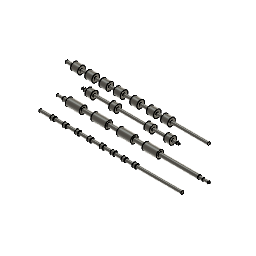
Salvage v1 (Autodesk Fusion 360 design; units mm, degrees)
Autodesk Fusion 360 part; units mm, degrees
sketch "Sketch1" plane through (0, 0, 0) normal (0, 1, 0) x (1, 0, 0) in component "axle1"
  line L0 (-152.5538, -2) -> (147.4462, -2)
  line L1 (147.4462, -2) -> (147.4462, -5)
  line L2 (147.4462, -5) -> (-152.5538, -5)
  line L3 (-152.5538, -5) -> (-152.5538, -2)
  line L4 (-136.5538, -5) -> (-121.5538, -5)
  line L5 (-121.5538, -5) -> (-121.5538, -10)
  line L6 (-121.5538, -10) -> (-136.5538, -10)
  line L7 (-136.5538, -10) -> (-136.5538, -5)
  line L8 (-106.5538, -5) -> (-91.5538, -5)
  line L9 (-91.5538, -5) -> (-91.5538, -10)
  line L10 (-91.5538, -10) -> (-106.5538, -10)
  line L11 (-106.5538, -10) -> (-106.5538, -5)
  line L12 (-76.5538, -5) -> (-61.5538, -5)
  line L13 (-61.5538, -5) -> (-61.5538, -10)
  line L14 (-61.5538, -10) -> (-76.5538, -10)
  line L15 (-76.5538, -10) -> (-76.5538, -5)
  line L16 (-46.5538, -5) -> (-31.5538, -5)
  line L17 (-31.5538, -5) -> (-31.5538, -10)
  line L18 (-31.5538, -10) -> (-46.5538, -10)
  line L19 (-46.5538, -10) -> (-46.5538, -5)
  line L20 (-11.5538, -5) -> (3.4462, -5)
  line L21 (3.4462, -5) -> (3.4462, -10)
  line L22 (3.4462, -10) -> (-11.5538, -10)
  line L23 (-11.5538, -10) -> (-11.5538, -5)
  line L24 (23.4462, -5) -> (38.4462, -5)
  line L25 (38.4462, -5) -> (38.4462, -10)
  line L26 (38.4462, -10) -> (23.4462, -10)
  line L27 (23.4462, -10) -> (23.4462, -5)
  line L28 (53.4462, -5) -> (68.4462, -5)
  line L29 (68.4462, -5) -> (68.4462, -10)
  line L30 (68.4462, -10) -> (53.4462, -10)
  line L31 (53.4462, -10) -> (53.4462, -5)
  dimension "d1" = 16
  dimension "d2" = 3
  dimension "d3" = 15
  dimension "d4" = 5
  dimension "d5" = 300
  dimension "d6" = 15
  dimension "d7" = 15
  dimension "d8" = 15
  dimension "d9" = 20
  dimension "d10" = 20
  dimension "d11" = 15
  constraint horizontal L0
  constraint vertical L1
  constraint horizontal L2
  constraint vertical L3
  constraint horizontal L4
  constraint vertical L5
  constraint horizontal L6
  constraint vertical L7
  constraint coincident L2 L4.start
  constraint horizontal L8
  constraint vertical L9
  constraint horizontal L10
  constraint vertical L11
  constraint coincident L2 L8.start
  constraint horizontal L12
  constraint vertical L13
  constraint horizontal L14
  constraint vertical L15
  constraint coincident L2 L12.start
  constraint horizontal L16
  constraint vertical L17
  constraint horizontal L18
  constraint vertical L19
  constraint coincident L2 L16.start
  constraint horizontal L20
  constraint vertical L21
  constraint horizontal L22
  constraint vertical L23
  constraint coincident L2 L20.start
  constraint horizontal L24
  constraint vertical L25
  constraint horizontal L26
  constraint vertical L27
  constraint coincident L2 L24.start
  constraint horizontal L28
  constraint vertical L29
  constraint horizontal L30
  constraint vertical L31
  constraint coincident L2 L28.start
  constraint equal L26 L30
  constraint equal L22 L26
  constraint equal L18 L22
  constraint equal L14 L18
  constraint equal L10 L14
  constraint equal L6 L10
  constraint equal L7 L11
  constraint equal L11 L15
  constraint equal L15 L19
  constraint equal L19 L23
  constraint equal L23 L27
  constraint equal L27 L31
  measures "d1" distance of L2.end L4.start
  measures "d2" distance of L0.start L2.end
  measures "d3" distance of L5.end L6.end
  measures "d4" distance of L4.start L6.end
  measures "d5" distance of L1.end L2.end
  measures "d6" distance of L4.end L8.start
  measures "d7" distance of L8.end L12.start
  measures "d8" distance of L12.end L16.start
  measures "d9" distance of L16.end L20.start
  measures "d10" distance of L20.end L24.start
  measures "d11" distance of L24.end L28.start
revolve "Revolve1" add sketch "Sketch1" angle 360 about axis through (-152.5538, 0, 2) along (1, 0, 0) makes body 1 in component "axle1"
sketch "Sketch1 (2)" plane through (0, 0, 0) normal (0, 1, 0) x (1, 0, 0) in component "axle2"
  line L0 (-92.2895, -1.3003) -> (207.7105, -1.3003)
  line L1 (207.7105, -1.3003) -> (207.7105, -4.3003)
  line L2 (207.7105, -4.3003) -> (-92.2895, -4.3003)
  line L3 (-92.2895, -4.3003) -> (-92.2895, -1.3003)
  line L4 (-67.2895, -4.3003) -> (-61.2895, -4.3003)
  line L5 (-61.2895, -4.3003) -> (-61.2895, -5.8003)
  line L6 (-61.2895, -5.8003) -> (-67.2895, -5.8003)
  line L7 (-67.2895, -5.8003) -> (-67.2895, -4.3003)
  line L8 (-41.2895, -4.3003) -> (-35.2895, -4.3003)
  line L9 (-35.2895, -4.3003) -> (-35.2895, -5.8003)
  line L10 (-35.2895, -5.8003) -> (-41.2895, -5.8003)
  line L11 (-41.2895, -5.8003) -> (-41.2895, -4.3003)
  line L12 (-15.2895, -4.3003) -> (-9.2895, -4.3003)
  line L13 (-9.2895, -4.3003) -> (-9.2895, -5.8003)
  line L14 (-9.2895, -5.8003) -> (-15.2895, -5.8003)
  line L15 (-15.2895, -5.8003) -> (-15.2895, -4.3003)
  line L16 (10.7105, -4.3003) -> (16.7105, -4.3003)
  line L17 (16.7105, -4.3003) -> (16.7105, -5.8003)
  line L18 (16.7105, -5.8003) -> (10.7105, -5.8003)
  line L19 (10.7105, -5.8003) -> (10.7105, -4.3003)
  line L20 (36.7105, -4.3003) -> (42.7105, -4.3003)
  line L21 (42.7105, -4.3003) -> (42.7105, -5.8003)
  line L22 (42.7105, -5.8003) -> (36.7105, -5.8003)
  line L23 (36.7105, -5.8003) -> (36.7105, -4.3003)
  line L24 (59.7105, -4.3003) -> (65.7105, -4.3003)
  line L25 (65.7105, -4.3003) -> (65.7105, -5.8003)
  line L26 (65.7105, -5.8003) -> (59.7105, -5.8003)
  line L27 (59.7105, -5.8003) -> (59.7105, -4.3003)
  line L28 (82.7105, -4.3003) -> (88.7105, -4.3003)
  line L29 (88.7105, -4.3003) -> (88.7105, -5.8003)
  line L30 (88.7105, -5.8003) -> (82.7105, -5.8003)
  line L31 (82.7105, -5.8003) -> (82.7105, -4.3003)
  line L32 (105.7105, -4.3003) -> (111.7105, -4.3003)
  line L33 (111.7105, -4.3003) -> (111.7105, -5.8003)
  line L34 (111.7105, -5.8003) -> (105.7105, -5.8003)
  line L35 (105.7105, -5.8003) -> (105.7105, -4.3003)
  dimension "d13" = 3
  dimension "d14" = 300
  dimension "d15" = 25
  dimension "d16" = 1.5
  dimension "d17" = 6
  dimension "d18" = 20
  dimension "d19" = 20
  dimension "d20" = 20
  dimension "d21" = 20
  dimension "d22" = 17
  dimension "d23" = 17
  dimension "d24" = 17
  constraint horizontal L0
  constraint vertical L1
  constraint horizontal L2
  constraint vertical L3
  constraint horizontal L4
  constraint vertical L5
  constraint horizontal L6
  constraint vertical L7
  constraint coincident L2 L4.start
  constraint horizontal L8
  constraint vertical L9
  constraint horizontal L10
  constraint vertical L11
  constraint coincident L2 L8.start
  constraint horizontal L12
  constraint vertical L13
  constraint horizontal L14
  constraint vertical L15
  constraint coincident L2 L12.start
  constraint horizontal L16
  constraint vertical L17
  constraint horizontal L18
  constraint vertical L19
  constraint coincident L2 L16.start
  constraint horizontal L20
  constraint vertical L21
  constraint horizontal L22
  constraint vertical L23
  constraint coincident L2 L20.start
  constraint horizontal L24
  constraint vertical L25
  constraint horizontal L26
  constraint vertical L27
  constraint coincident L2 L24.start
  constraint horizontal L28
  constraint vertical L29
  constraint horizontal L30
  constraint vertical L31
  constraint coincident L2 L28.start
  constraint horizontal L32
  constraint vertical L33
  constraint horizontal L34
  constraint vertical L35
  constraint coincident L2 L32.start
  constraint equal L6 L10
  constraint equal L10 L14
  constraint equal L14 L18
  constraint equal L18 L22
  constraint equal L22 L26
  constraint equal L26 L30
  constraint equal L30 L34
  constraint equal L31 L35
  constraint equal L27 L31
  constraint equal L23 L27
  constraint equal L19 L23
  constraint equal L15 L19
  constraint equal L11 L15
  constraint equal L7 L11
  measures "d13" distance of L0.start L2.end
  measures "d14" distance of L1.end L2.end
  measures "d15" distance of L2.end L4.start
  measures "d16" distance of L4.start L6.end
  measures "d17" distance of L5.end L6.end
  measures "d18" distance of L4.end L8.start
  measures "d19" distance of L8.end L12.start
  measures "d20" distance of L12.end L16.start
  measures "d21" distance of L16.end L20.start
  measures "d22" distance of L20.end L24.start
  measures "d23" distance of L24.end L28.start
  measures "d24" distance of L28.end L32.start
revolve "Revolve1'" add sketch "Sketch1 (2)" angle 360 about axis through (-92.2895, 0, 1.3003) along (1, 0, 0) separate body makes body 2 in component "axle2"
sketch "Sketch1 (3)" plane through (0, 0, 0) normal (0, 1, 0) x (1, 0, 0) in component "axle3"
  line L0 (224.232, -5.3472) -> (-61.268, -5.3472)
  line L1 (-61.768, -4.8472) -> (-61.768, -3.6472)
  line L2 (-50.768, -5.3472) -> (-20.768, -5.3472)
  line L3 (-20.768, -5.3472) -> (-20.768, -9.1472)
  line L4 (-20.768, -9.1472) -> (-50.768, -9.1472)
  line L5 (-50.768, -9.1472) -> (-50.768, -5.3472)
  line L6 (3.232, -5.3472) -> (33.232, -5.3472)
  line L7 (33.232, -5.3472) -> (33.232, -9.1472)
  line L8 (33.232, -9.1472) -> (3.232, -9.1472)
  line L9 (3.232, -9.1472) -> (3.232, -5.3472)
  line L10 (57.232, -5.3472) -> (87.232, -5.3472)
  line L11 (87.232, -5.3472) -> (87.232, -9.1472)
  line L12 (87.232, -9.1472) -> (57.232, -9.1472)
  line L13 (57.232, -9.1472) -> (57.232, -5.3472)
  line L14 (111.232, -5.3472) -> (141.232, -5.3472)
  line L15 (141.232, -5.3472) -> (141.232, -9.1472)
  line L16 (141.232, -9.1472) -> (111.232, -9.1472)
  line L17 (111.232, -9.1472) -> (111.232, -5.3472)
  line L18 (-61.768, -3.6472) -> (-75.193, -3.6472)
  line L19 (-75.768, -3.0722) -> (-75.768, -1.3472)
  line L20 (224.232, -5.3472) -> (224.232, -1.3472)
  line L21 (224.232, -1.3472) -> (-75.768, -1.3472)
  line L22 (224.232, -4.3472) -> (232.962, -4.3472)
  line L23 (233.462, -3.8472) -> (233.462, -1.3472)
  line L24 (233.462, -1.3472) -> (224.232, -1.3472)
  line L25 (224.232, -1.3472) -> (224.232, -4.3472)
  line L26 (233.462, -3.8472) -> (244.212, -3.8472)
  line L27 (245.962, -2.8472) -> (245.962, -1.3472)
  line L28 (245.962, -1.3472) -> (233.462, -1.3472)
  line L29 (233.462, -1.3472) -> (233.462, -3.8472)
  line L30 (-75.193, -3.6472) -> (-75.768, -3.0722)
  line L31 (-61.268, -5.3472) -> (-61.768, -4.8472)
  line L32 (244.212, -3.8472) -> (245.962, -2.8472)
  line L33 (232.962, -4.3472) -> (233.462, -3.8472)
  point P0 (-61.768, -5.3472)
  point P1 (-75.768, -3.6472)
  point P2 (233.462, -4.3472)
  point P3 (245.962, -3.8472)
  dimension "d26" = 14
  dimension "d27" = 2.3
  dimension "d29" = 3.8
  dimension "d30" = 30
  dimension "d32" = 11
  dimension "d33" = 24
  dimension "d34" = 24
  dimension "d35" = 24
  dimension "d36" = 300
  dimension "d37" = 2.5
  dimension "d38" = 3
  dimension "d39" = 4
  dimension "d40" = 0.575
  dimension "d41" = 45
  dimension "d42" = 0.5
  dimension "d43" = 45
  dimension "d44" = 9.23
  dimension "d45" = 12.5
  dimension "d46" = 1.75
  dimension "d47" = 1
  dimension "d48" = 0.5
  dimension "d49" = 0.5
  constraint horizontal L0
  constraint vertical L1
  constraint horizontal L2
  constraint vertical L3
  constraint horizontal L4
  constraint vertical L5
  constraint coincident L0 L2.start
  constraint horizontal L6
  constraint vertical L7
  constraint horizontal L8
  constraint vertical L9
  constraint coincident L0 L6.start
  constraint horizontal L10
  constraint vertical L11
  constraint horizontal L12
  constraint vertical L13
  constraint coincident L0 L10.start
  constraint horizontal L14
  constraint vertical L15
  constraint horizontal L16
  constraint vertical L17
  constraint coincident L0 L14.start
  constraint horizontal L18
  constraint vertical L19
  constraint equal L12 L16
  constraint equal L8 L12
  constraint equal L4 L8
  constraint equal L5 L9
  constraint equal L13 L17
  constraint equal L9 L13
  constraint perpendicular L19 L21
  constraint horizontal L22
  constraint vertical L23
  constraint horizontal L24
  constraint vertical L25
  constraint coincident L20 L22.start
  constraint horizontal L26
  constraint vertical L27
  constraint horizontal L28
  constraint vertical L29
  constraint collinear L24 L28
  constraint collinear L21 L24
  constraint coincident P1 L18
  constraint coincident P1 L19
  constraint coincident P0 L0
  constraint coincident P0 L1
  constraint collinear L23 L29
  constraint coincident P3 L26
  constraint coincident P3 L27
  constraint coincident P2 L22
  constraint coincident P2 L23
  measures "d26" distance of L1.end P1
  measures "d27" distance of P1 L19.end
  measures "d29" distance of L2.start L4.end
  measures "d30" distance of L3.end L4.end
  measures "d32" distance of P0 L2.start
  measures "d33" distance of L2.end L6.start
  measures "d34" distance of L6.end L10.start
  measures "d35" distance of L10.end L14.start
  measures "d36" distance of L19.end L20.end
  measures "d37" distance of P3 L27.end
  measures "d38" distance of P2 L23.end
  measures "d39" distance of L20.end L0.start
  measures "d40" distance of P1 L18.end
  measures "d41" angle of L18 L30
  measures "d42" distance of P0 L0.end
  measures "d43" angle of L0 L31
  measures "d44" distance of L22.start P2
  measures "d45" distance of L23.start P3
  measures "d46" distance of P3 L26.end
  measures "d47" distance of P3 L27.start
  measures "d48" distance of P2 L22.end
  measures "d49" distance of P2 L23.start
revolve "Revolve1''" add sketch "Sketch1 (3)" angle 360 about axis through (245.962, 0, 1.3472) along (-1, 0, 0) separate body makes body 3 in component "axle3"
copy_body "CutPasteBodies1" bodies 3 removing the originals makes body 4 in component "axle3"
sketch "Sketch1 (4)" plane through (0, 0, 0) normal (1, 0, 0) x (0, 1, 0) in component "axle4"
  line L0 (-204.9118, 10.3817) -> (-8.8818, 10.3817)
  line L1 (-8.8818, 10.3817) -> (-8.8818, 12.8817)
  line L2 (-9.3818, 13.3817) -> (-204.4118, 13.3817)
  line L3 (-17.6918, 13.3817) -> (-29.2918, 13.3817)
  line L4 (-29.2918, 13.3817) -> (-29.2918, 18.2617)
  line L5 (-29.2918, 18.2617) -> (-17.6918, 18.2617)
  line L6 (-17.6918, 18.2617) -> (-17.6918, 13.3817)
  line L7 (-67.5118, 13.3817) -> (-79.1118, 13.3817)
  line L8 (-79.1118, 13.3817) -> (-79.1118, 18.2617)
  line L9 (-79.1118, 18.2617) -> (-67.5118, 18.2617)
  line L10 (-67.5118, 18.2617) -> (-67.5118, 13.3817)
  line L11 (-142.1118, 13.3817) -> (-153.7118, 13.3817)
  line L12 (-153.7118, 13.3817) -> (-153.7118, 18.2617)
  line L13 (-153.7118, 18.2617) -> (-142.1118, 18.2617)
  line L14 (-142.1118, 18.2617) -> (-142.1118, 13.3817)
  line L15 (-183.7118, 13.3817) -> (-195.3118, 13.3817)
  line L16 (-195.3118, 13.3817) -> (-195.3118, 18.2617)
  line L17 (-195.3118, 18.2617) -> (-183.7118, 18.2617)
  line L18 (-183.7118, 18.2617) -> (-183.7118, 13.3817)
  line L19 (-204.9118, 10.3817) -> (-208.9118, 10.3817)
  line L20 (-208.9118, 10.3817) -> (-208.9118, 11.6817)
  line L21 (-208.4118, 12.1817) -> (-204.9118, 12.1817)
  line L22 (-204.9118, 12.1817) -> (-204.9118, 10.3817)
  line L23 (-8.8818, 12.3817) -> (-4.8618, 12.3817)
  line L24 (-4.3618, 11.8817) -> (-4.3618, 10.3817)
  line L25 (-4.3618, 10.3817) -> (-8.8818, 10.3817)
  line L26 (-8.8818, 10.3817) -> (-8.8818, 12.3817)
  line L27 (-204.9118, 12.1817) -> (-204.9118, 12.8817)
  line L28 (-8.8818, 12.8817) -> (-9.3818, 13.3817)
  line L29 (-4.8618, 12.3817) -> (-4.3618, 11.8817)
  line L30 (-208.9118, 11.6817) -> (-208.4118, 12.1817)
  line L31 (-204.4118, 13.3817) -> (-204.9118, 12.8817)
  point P0 (-8.8818, 13.3817)
  point P1 (-204.9118, 13.3817)
  point P2 (-208.9118, 12.1817)
  point P3 (-4.3618, 12.3817)
  dimension "d52" = 4.52
  dimension "d53" = 2
  dimension "d54" = 3
  dimension "d55" = 1.8
  dimension "d57" = 4.88
  dimension "d58" = 11.6
  dimension "d59" = 4
  dimension "d60" = 9.6
  dimension "d61" = 30
  dimension "d62" = 63
  dimension "d63" = 38.22
  dimension "d64" = 8.81
  dimension "d65" = 0.5
  dimension "d66" = 45
  dimension "d67" = 0.5
  dimension "d68" = 45
  dimension "d69" = 0.5
  dimension "d70" = 45
  dimension "d71" = 0.5
  dimension "d72" = 45
  constraint horizontal L0
  constraint vertical L1
  constraint horizontal L2
  constraint horizontal L3
  constraint vertical L4
  constraint horizontal L5
  constraint vertical L6
  constraint coincident L2 L3.start
  constraint horizontal L7
  constraint vertical L8
  constraint horizontal L9
  constraint vertical L10
  constraint coincident L2 L7.start
  constraint horizontal L11
  constraint vertical L12
  constraint horizontal L13
  constraint vertical L14
  constraint coincident L2 L11.start
  constraint horizontal L15
  constraint vertical L16
  constraint horizontal L17
  constraint vertical L18
  constraint coincident L2 L15.start
  constraint horizontal L19
  constraint vertical L20
  constraint horizontal L21
  constraint vertical L22
  constraint horizontal L23
  constraint vertical L24
  constraint horizontal L25
  constraint vertical L26
  constraint coincident L1 L23.start
  constraint collinear L0 L25
  constraint perpendicular L15 L27
  constraint equal L6 L10
  constraint equal L10 L14
  constraint equal L14 L18
  constraint equal L5 L9
  constraint equal L9 L13
  constraint equal L13 L17
  constraint coincident P0 L1
  constraint coincident P0 L2
  constraint coincident P3 L23
  constraint coincident P3 L24
  constraint coincident P2 L20
  constraint coincident P2 L21
  constraint coincident P1 L2
  constraint coincident P1 L27
  measures "d52" distance of L24.end L0.end
  measures "d53" distance of P3 L24.end
  measures "d54" distance of L0.end P0
  measures "d55" distance of L19.end P2
  measures "d57" distance of L3.start L5.end
  measures "d58" distance of L4.end L5.end
  measures "d59" distance of L0.start L19.end
  measures "d60" distance of P1 L15.end
  measures "d61" distance of L11.end L15.start
  measures "d62" distance of L7.end L11.start
  measures "d63" distance of L3.end L7.start
  measures "d64" distance of P0 L3.start
  measures "d65" distance of P0 L1.end
  measures "d66" angle of L1 L28
  measures "d67" distance of P3 L23.end
  measures "d68" angle of L23 L29
  measures "d69" distance of P2 L20.end
  measures "d70" angle of L20 L30
  measures "d71" distance of P1 L2.end
  measures "d72" angle of L2 L31
revolve "Revolve1'''" add sketch "Sketch1 (4)" angle 360 about axis through (0, -204.9118, 10.3817) along (0, 1, 0) separate body makes body 5 in component "axle4"
move_face "MoveFace1" to x (0, 0, -1) y (0, 1, 0) z (1, 0, 0) at (-10.3817, 0, 10.3817) 1 faces at (-0.2987, -42.0318, 13.3668) on bodies 5 in component "axle4"
move_body "Move1" bodies 5 to x (1, 0, 0) y (0, 1, 0) z (0, 0, 1) at (-3.9782, 0, -8.6193) in component "axle4"
component "axle1" placed x (1, 0, 0) y (0, 1, 0) z (0, 0, 1) at (0, 0, 0)
component "axle2" placed x (1, 0, 0) y (0, 1, 0) z (0, 0, 1) at (0.4799, -116.7215, 0)
component "axle3" placed x (1, 0, 0) y (0, 1, 0) z (0, 0, 1) at (-26.8349, -70.2825, 0)
component "axle4" placed x (0, 1, 0) y (-1, 0, 0) z (0, 0, 1) at (-91.7813, -28.0002, 0)
equation "d16 = ( 3 / 2 ) * 1 mm"
equation "d27 = ( 4.6 / 2 ) * 1 mm"
equation "d37 = ( 5 / 2 ) * 1 mm"
equation "d49 = d48"
equation "d55 = ( 3.6 / 2 ) * 1 mm"
